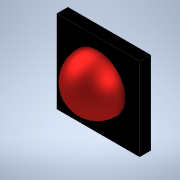
# Autodesk Inventor part: BUTTON
Saved by Autodesk Inventor 2021 (Build 250183000, 183)
## iProperties
Created: 2021-07-04
Part Number: BUTTON
Material: Generic
Document SubType Name: Modeling
Designer: Manojgouda K R
Density: 1 g/cm^3
Appearance: Default
Author: Manojgouda K R
Autodesk Inventor part; units mm, degrees
ref_plane "YZ Plane" through (0, 0, 0) normal (1, 0, 0) x (0, 1, 0)
ref_plane "XZ Plane" through (0, 0, 0) normal (0, 1, 0) x (-1, 0, 0)
ref_plane "XY Plane" through (0, 0, 0) normal (0, 0, 1) x (1, 0, 0)
sketch "Sketch1" plane through (0, 0, 0) normal (0, 0, 1) x (1, 0, 0)
  line L0 (-3.9316, 1.4634) -> (-2.4316, 1.4634)
  line L1 (-2.4316, 1.4634) -> (-2.4316, -0.0366)
  line L2 (-2.4316, -0.0366) -> (-3.9316, -0.0366)
  line L3 (-3.9316, -0.0366) -> (-3.9316, 1.4634)
  point P0 (0, 0)
  dimension "d0" = 1.5
  dimension "d1" = 1.5
  constraints: 8 end point, 2 parallel, 1 horizontal, 1 perpendicular
  measures "d0" distance of L1.end L2.end
  measures "d1" distance of L0.end L1.end
extrude "Extrusion1" add sketch "Sketch1" along normal blind 0.2
sketch "Sketch2" plane through (0, 0, 0.2) normal (0, 0, 1) x (1, 0, 0)
  arc A0 (-2.8652, 0.378) -> (-3.5209, 1.133) centre (-3.1933, 0.7553) ccw
  line L0 (-3.5209, 1.133) -> (-2.8652, 0.378)
  point P0 (0, 0)
  dimension "d6" = 1
  constraints: 2 end point, 2 point on circle, 1 centre point
  measures "d6" diameter of A0
revolve "Revolution1" add sketch "Sketch2" angle 180 about axis through (-3.5209, 1.133, 0.2) along (0.6557, -0.755, 0)
body "Solid1"
